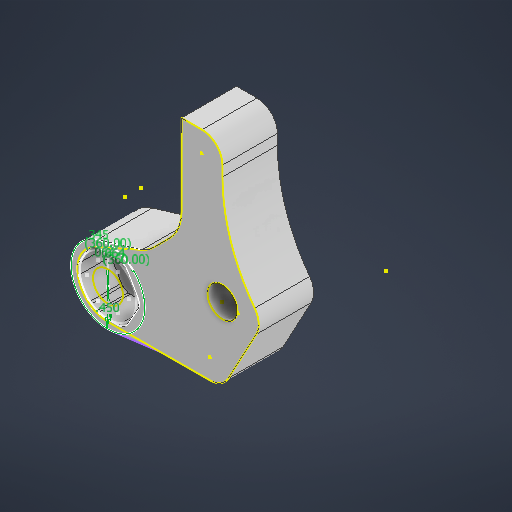
# Autodesk Inventor part: Goal Jaw Tooth Straight'
Saved by Autodesk Inventor 2025 (Build 290162000, 162)
## iProperties
Created: 2025-02-08
Part Number: Goal Jaw Tooth Straight'
Material: Generic
Document SubType Name: Modeling
Designer: Juan
Density: 1 g/cm^3
Appearance: Default
Author: Juan
Autodesk Inventor part; units mm, degrees
ref_plane "YZ Plane" through (0, 0, 0) normal (1, 0, 0) x (0, 1, 0)
ref_plane "XZ Plane" through (0, 0, 0) normal (0, 1, 0) x (-1, 0, 0)
ref_plane "XY Plane" through (0, 0, 0) normal (0, 0, 1) x (1, 0, 0)
sketch "Sketch1" plane through (0, 0, 0) normal (0, 0, 1) x (1, 0, 0)
  circle A0 centre (0, 0) radius 2.3241
  circle A1 centre (0, 0) radius 11.5062
  line L0 (0, 0) -> (0, 6.35)
  line L1 (0, 6.35) -> (1.470802, 6.35)
  line L2 (1.470802, 6.35) -> (9.595319, 6.35)
  line L3 (0, 6.35) -> (0, 21.59)
  line L4 (0, 21.59) -> (-6.35, 21.59)
  line L5 (0, 6.35) -> (-35.466264, 6.35)
  line L6 (-30.570655, -30.094759) -> (-7.749339, -41.24588)
  circle A2 centre (4.797659, -18.435969) radius 2.3241
  circle A3 centre (4.797659, -18.435969) radius 4.7625
  line L7 (4.797659, -18.435969) -> (-17.78874, -6.816393)
  circle A4 centre (-17.78874, -6.816393) radius 2.3241
  circle A5 centre (-17.78874, -6.816393) radius 4.7625
  line L8 (0, 6.35) -> (-19.731915, -2.46835)
  line L9 (9.595319, 6.35) -> (0, -11.5062)
  line L10 (0, -11.5062) -> (-17.769268, -11.578853)
  line L11 (-6.35, 21.59) -> (-6.35, 6.35)
  line L12 (-6.35, 6.35) -> (-11.439446, 1.23762)
  line L13 (0, 6.35) -> (6.251202, 0.12684)
  dimension "d0" = 4.6482
  dimension "d1" = 23.0124
  dimension "d2" = 6.35
  dimension "d3" = 15.24
  dimension "d4" = 6.35
  dimension "d5" = 25.4
  dimension "d6" = 4.6482
  dimension "d7" = 9.525
  dimension "d8" = 25.4
  dimension "d9" = 4.6482
  dimension "d10" = 9.525
  constraints: 28 end point, 6 centre point, 5 coincident, 5 point on circle, 5 point on line, 3 perpendicular, 2 tangent, 1 horizontal, 1 vertical
  measures "d0" diameter of A0
  measures "d1" diameter of A1
  measures "d2" distance of L0.start L0.end
  measures "d3" distance of L0.end L3.end
  measures "d4" distance of L3.end L4.end
  measures "d5" distance of L6.start L6.end
  measures "d6" diameter of A2
  measures "d7" diameter of A3
  measures "d8" distance of L7.start L7.end
  measures "d9" diameter of A4
  measures "d10" diameter of A5
extrude "Extrusion2" add sketch "Sketch1" along normal blind 5.999988 contours L10 L7 A5 L8 A1 | A1 L8 L13 L9 | L3 L5 L11 A1 | A1 L11 L4 L3 | L12 L5 L8 | L10 A5 L7 | A5
fillet "Fillet3" radius 25.4 1 edges at (0, 6.35, 3)
fillet "Fillet4" radius 3.175 1 edges at (6.2512, 0.1268, 3)
fillet "Fillet5" radius 3.175 1 edges at (0, -11.5062, 3)
fillet "Fillet6" radius 3.175 1 edges at (0, 21.59, 3)
fillet "Fillet7" radius 6.35 2 edges at (-6.35, 6.35, 3) (-11.4394, 1.2376, 3)
sketch "Sketch2" plane through (0, 0, 5.999988) normal (0, 0, 1) x (1, 0, 0)
  arc A0 (0, 18.415) -> (-3.175, 21.59) centre (-3.175, 18.415) ccw
  line L0 (-3.175, 21.59) -> (-6.35, 21.59)
  line L1 (-6.35, 21.59) -> (-6.35, 8.971898)
  arc A1 (-8.19979, 4.491875) -> (-6.35, 8.971898) centre (-12.7, 8.971898) ccw
  line L2 (-8.19979, 4.491875) -> (-10.60716, 2.073657)
  arc A2 (-12.51647, 0.75629) -> (-10.60716, 2.073657) centre (-15.10737, 6.55368) ccw
  line L3 (-12.51647, 0.75629) -> (-19.731915, -2.46835)
  arc A3 (-19.731915, -2.46835) -> (-17.769268, -11.578853) centre (-17.78874, -6.816393) ccw
  line L4 (-17.769268, -11.578853) -> (-1.889423, -11.513925)
  arc A4 (-1.889423, -11.513925) -> (0.894369, -9.841843) centre (-1.902404, -8.338952) ccw
  line L5 (0.894369, -9.841843) -> (5.256051, -1.725065)
  arc A5 (5.256051, -1.725065) -> (5.008247, 1.670809) centre (2.459278, -0.222173) ccw
  arc A6 (0, 16.814666) -> (5.008247, 1.670809) centre (25.4, 16.814666) ccw
  line L6 (0, 16.814666) -> (0, 18.415)
  circle A7 centre (-17.78874, -6.816393) radius 2.3241
  circle A8 centre (0, 0) radius 2.3241
  circle A9 centre (-17.78874, -6.816393) radius 4.3815
  line L7 (-17.78874, -6.816393) -> (-17.78874, -2.434893)
  line L8 (-17.78874, -2.434893) -> (-16.17584, -2.434893)
  line L9 (-17.78874, -2.434893) -> (-19.40164, -2.434893)
  line L10 (-21.583231, -4.625643) -> (-20.776781, -3.228831)
  line L11 (-21.583231, -4.625643) -> (-22.389681, -6.022456)
  line L12 (-21.583231, -9.007143) -> (-22.389681, -7.610331)
  line L13 (-21.583231, -9.007143) -> (-20.776781, -10.403956)
  line L14 (-17.78874, -11.197893) -> (-19.40164, -11.197893)
  line L15 (-17.78874, -11.197893) -> (-16.17584, -11.197893)
  line L16 (-13.99425, -9.007143) -> (-14.8007, -10.403956)
  line L17 (-13.99425, -9.007143) -> (-13.1878, -7.610331)
  line L18 (-13.99425, -4.625643) -> (-13.1878, -6.022456)
  line L19 (-13.99425, -4.625643) -> (-14.8007, -3.228831)
  arc A10 (-14.8007, -3.228831) -> (-16.17584, -2.434893) centre (-16.17584, -4.022768) ccw
  arc A11 (-19.40164, -2.434893) -> (-20.776781, -3.228831) centre (-19.40164, -4.022768) ccw
  arc A12 (-22.389681, -6.022456) -> (-22.389681, -7.610331) centre (-21.01454, -6.816393) ccw
  arc A13 (-20.776781, -10.403956) -> (-19.40164, -11.197893) centre (-19.40164, -9.610018) ccw
  arc A14 (-16.17584, -11.197893) -> (-14.8007, -10.403956) centre (-16.17584, -9.610018) ccw
  arc A15 (-13.1878, -7.610331) -> (-13.1878, -6.022456) centre (-14.56294, -6.816393) ccw
  circle A16 centre (-17.78874, -6.816393) radius 5.715
  line L20 (-12.51647, 0.75629) -> (-19.448583, -1.347742)
  line L21 (-9.597787, -11.545443) -> (-17.074988, -12.486647)
  point P0 (-19.737366, -11.161996)
  point P1 (-20.57783, -10.676754)
  point P2 (-22.526456, -7.301635)
  point P3 (-22.526456, -6.331151)
  point P4 (-20.57783, -2.956032)
  point P5 (-19.737366, -2.47079)
  dimension "d22" = 8.763
  dimension "d23" = 1.6129
  dimension "d24" = 1.6129
  dimension "d27" = 360
  dimension "d31" = 360
  dimension "d33" = 11.43
  constraints: 30 end point, 14 point on circle, 7 centre point, 7 point on line, 3 tangent, 2 coincident, 2 horizontal, 1 vertical, 1 vertical alignment, 58 other
  measures "d23" distance of L7.end L8.end
  measures "d24" distance of L7.end L9.end
  measures "d33" diameter of A16
extrude "Extrusion3" add sketch "Sketch2" against normal up to surface (5.999988 mm away) contours L3 A16 L20 | L21 A16 L4 | L3 A11 A3 A12 A13 L4 A16 | A3 A11 | A13 A3 | A3 A12
extrude "Extrusion5" cut sketch "Sketch2" against normal blind 5.08 contours A11 L9 A9 L10 A3 | A3 A11 | A3 A13 L13 A9 L14 | A12 L11 A9 L12 A3 | A3 A12 | L8 A10 L19 A9 | A9 | L18 A15 L17 A9 | A9 L16 A14 L15
sketch "Sketch3" plane through (0, 0, 0) normal (0, 0, -1) x (-1, 0, 0)
  circle A0 centre (0, 0) radius 2.3241
  circle A1 centre (17.78874, -6.816393) radius 2.3241
  arc A2 (3.175, 21.59) -> (0, 18.415) centre (3.175, 18.415) ccw
  line L0 (0, 16.814666) -> (0, 18.415)
  arc A3 (-5.008247, 1.670809) -> (0, 16.814666) centre (-25.4, 16.814666) ccw
  arc A4 (-5.008247, 1.670809) -> (-5.256051, -1.725065) centre (-2.459278, -0.222173) ccw
  line L1 (-0.894369, -9.841843) -> (-5.256051, -1.725065)
  arc A5 (-0.894369, -9.841843) -> (1.889423, -11.513925) centre (1.902404, -8.338952) ccw
  line L2 (9.597787, -11.545443) -> (1.889423, -11.513925)
  line L3 (9.597787, -11.545443) -> (17.074988, -12.486647)
  arc A6 (17.074988, -12.486647) -> (19.448583, -1.347742) centre (17.78874, -6.816393) ccw
  line L4 (19.448583, -1.347742) -> (12.51647, 0.75629)
  arc A7 (10.60716, 2.073657) -> (12.51647, 0.75629) centre (15.10737, 6.55368) ccw
  line L5 (8.19979, 4.491875) -> (10.60716, 2.073657)
  arc A8 (6.35, 8.971898) -> (8.19979, 4.491875) centre (12.7, 8.971898) ccw
  line L6 (6.35, 21.59) -> (6.35, 8.971898)
  line L7 (3.175, 21.59) -> (6.35, 21.59)
extrude "Extrusion6" add sketch "Sketch3" along normal blind 2.54
body "Solid2"
